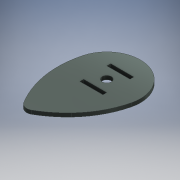
# Autodesk Inventor part: leva00
Saved by Autodesk Inventor 2016 (Build 200138000, 138)
## iProperties
Created: 2016-09-20
Part Number: leva00
Material: Madera (abedul)
Document SubType Name: Modeling
Designer: i95sa
Density: 0.55 g/cm^3
Appearance: Gris plomo - Pulido
Author: i95sa
Autodesk Inventor part; units mm, degrees
ref_plane "YZ Plane" through (0, 0, 0) normal (1, 0, 0) x (0, 1, 0)
ref_plane "XZ Plane" through (0, 0, 0) normal (0, 1, 0) x (-1, 0, 0)
ref_plane "XY Plane" through (0, 0, 0) normal (0, 0, 1) x (1, 0, 0)
sketch "Boceto1" plane through (0, 0, 0) normal (0, 0, 1) x (1, 0, 0)
  arc A0 (9.0361, 35.1935) -> (-9.0361, -35.1935) centre (0, 0) ccw
  arc A1 (-13.9059, -54.16) -> (-18.0764, -70.4031) centre (-15.9912, -62.2815) ccw
  line L0 (-18.6802, -72.7545) -> (-26.8018, -70.6693)
  line L1 (-35.084, 9.4524) -> (-48.6199, 12.9279)
  line L2 (-48.6199, 12.9279) -> (-26.8018, -70.6693)
  line L3 (-26.8018, -70.6693) -> (-35.2717, -38.2163)
  arc A2 (-35.084, 9.4524) -> (-35.2717, -38.2163) centre (54.6945, -14.7359) ccw
  arc A3 (-35.2717, -38.2163) -> (-23.1352, -66.6715) centre (66.3204, -11.7016) ccw
  line L4 (0.6951, 2.7072) -> (9.0361, 35.1935)
  line L5 (-0.6951, -2.7072) -> (-18.6802, -72.7545)
  arc A4 (-9.0361, -35.1935) -> (9.0361, 35.1935) centre (0, 0) ccw
  arc A5 (-18.0764, -70.4031) -> (-13.9059, -54.16) centre (-15.9912, -62.2815) ccw
  line L6 (-18.6802, -72.7545) -> (-10.5586, -74.8398)
  line L7 (35.298, -8.6186) -> (48.834, -12.0941)
  line L8 (48.834, -12.0941) -> (-10.5586, -74.8398)
  line L9 (-10.5586, -74.8398) -> (12.498, -50.4815)
  arc A6 (12.498, -50.4815) -> (35.298, -8.6186) centre (-55.0282, 13.4361) ccw
  arc A7 (-11.8457, -69.5701) -> (12.498, -50.4815) centre (-63.7543, 21.6959) ccw
  dimension "d0" = 72.67
  dimension "d6" = 16.77
  dimension "d7" = 8.385
  dimension "d8" = 13.975
  dimension "d9" = 33.54
  constraints: 20 end point, 20 point on circle, 8 centre point, 6 symmetric about line, 5 point on line, 4 tangent, 1 collinear, 4 other
  measures "d0" diameter of A0
  measures "d6" diameter of A1
  measures "d7" distance of L0.start L0.end
  measures "d8" distance of L1.start L1.end
  measures "d9" distance of L0.end L3.end
extrude "Extrusión2" add sketch "Boceto1" along normal blind 4 contours A4 A0 | A0 L5 A1 A3 A2 | A6 A7 A5 L5 A4 | L5 A1 | A5 L5
sketch "Boceto2" plane through (0, 0, 4) normal (0, 0, 1) x (1, 0, 0)
  line L0 (0, 0) -> (0, 12.5)
  line L1 (0, 12.5) -> (-12.5, 12.5)
  line L2 (-12.5, 12.5) -> (-12.5, 16.7)
  line L3 (-12.5, 16.7) -> (12.5, 16.7)
  line L4 (12.5, 16.7) -> (12.5, 12.5)
  line L5 (12.5, 12.5) -> (0, 12.5)
  line L6 (0, 0) -> (12.5, 0)
  line L7 (0, 0) -> (0, -12.5)
  line L8 (0, -12.5) -> (-12.5, -12.5)
  line L9 (-12.5, -12.5) -> (-12.5, -16.7)
  line L10 (-12.5, -16.7) -> (12.5, -16.7)
  line L11 (12.5, -16.7) -> (12.5, -12.5)
  line L12 (12.5, -12.5) -> (0, -12.5)
  circle A0 centre (0, 0) radius 5
  dimension "d24" = 12.5
  dimension "d25" = 12.5
  dimension "d26" = 4.2
  dimension "d27" = 25
  dimension "d28" = 10
  constraints: 26 end point, 5 perpendicular, 5 symmetric about line, 3 point on line, 1 centre point, 1 coincident, 1 parallel, 1 vertical
  measures "d24" distance of L0.start L0.end
  measures "d25" distance of L0.end L1.end
  measures "d26" distance of L1.end L2.end
  measures "d27" distance of L2.end L3.end
  measures "d28" diameter of A0
extrude "Extrusión3" cut sketch "Boceto2" against normal blind 4
